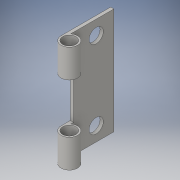
# Autodesk Inventor part: Hinge Wall 1
Saved by Autodesk Inventor 2016 (Build 200138000, 138)
## iProperties
Created: 2016-04-01
Part Number: Hinge Wall 1
Material: Generic
Document SubType Name: Modeling
Designer: amycroft3
Density: 1 g/cm^3
Appearance: Default
Author: amycroft3
Autodesk Inventor part; units mm, degrees
ref_plane "YZ Plane" through (0, 0, 0) normal (1, 0, 0) x (0, 1, 0)
ref_plane "XY Plane" through (0, 0, 0) normal (0, 0, 1) x (1, 0, 0)
sketch "Sketch1" plane through (0, 0, 0) normal (0, 1, 0) x (-1, 0, 0)
  circle A0 centre (0, 0) radius 2.3876
  arc A1 (2.9591, 0) -> (1.8161, -2.3362) centre (0, 0) ccw
  line L0 (2.9591, 0) -> (2.3876, 0)
  line L1 (1.8161, -2.3362) -> (1.8161, -17.78)
  line L2 (1.8161, -17.78) -> (2.9591, -17.78)
  line L3 (2.9591, -17.78) -> (2.9591, 0)
  dimension "d0" = 4.7752
  dimension "d1" = 5.9182
  dimension "d2" = 17.78
  dimension "d3" = 1.143
  constraints: 8 end point, 2 coincident, 2 parallel, 2 point on circle, 1 centre point, 1 horizontal, 1 horizontal alignment, 1 perpendicular, 1 tangent, 2 other
  measures "d1" diameter of A1
  measures "d2" distance of L2.end L0.start
  measures "d3" distance of L1.end L2.end
extrude "Extrusion1" add sketch "Sketch1" along normal blind 38.1
ref_plane "Work Plane1" through (0, 10.16, 0) normal (0, 1, 0) x (-1, 0, 0)
sketch "Sketch2" plane through (0, 10.16, 0) normal (0, 1, 0) x (-1, 0, 0)
  circle A0 centre (0, 0) radius 2.3876 projected
  arc A1 (2.9591, 0) -> (1.8161, -2.3362) centre (0, 0) ccw projected
  line L0 (1.8161, -2.3362) -> (1.8161, -17.78) projected
  line L1 (1.8161, -17.78) -> (2.9591, -17.78) projected
  line L2 (2.9591, -17.78) -> (2.9591, 0) projected
  line L3 (2.9591, 3.4646) -> (-3.1409, 3.4646)
  line L4 (-3.1409, 3.4646) -> (-3.1409, -3.337)
  line L5 (-3.1409, -3.337) -> (2.9591, -3.337)
  line L6 (2.9591, -3.337) -> (2.9591, 3.4646)
  dimension "d7" = 0
  dimension "d8" = 6.1
  dimension "d9" = 21.2446
  dimension "d10" = 14.443
  constraints: 8 end point, 2 parallel, 1 horizontal, 1 perpendicular
  measures "d7" distance between parallel lines of L2 L6
  measures "d8" distance between parallel lines of L2 L4
  measures "d9" distance between parallel lines of L1 L3
  measures "d10" distance between parallel lines of L1 L5
extrude "Extrusion2" cut sketch "Sketch2" along normal blind 17.78 contours L2 L5 L0 A1 | A1 L0 L5 L4 L3 L6
sketch "Sketch3" plane through (-1.8161, 0, -2.3362) normal (1, 0, 0) x (0, 0, -1)
  circle A0 centre (9.0938, 5.08) radius 2.54
  circle A1 centre (9.0938, 33.02) radius 2.54
  line L0 (15.4438, 0) -> (15.4438, 38.1) projected
  line L1 (0, 0) -> (15.4438, 0) projected
  line L2 (0, 38.1) -> (15.4438, 38.1) projected
  point P0 (-2.3362, 0)
  dimension "d13" = 6.35
  dimension "d14" = 5.08
  dimension "d15" = 5.08
  dimension "d17" = 5.08
  constraints: 2 centre point, 1 equal radius, 1 vertical alignment
  measures "d13" distance from line of A0.centre L0
  measures "d14" distance from line of A0.centre L1
  measures "d15" diameter of A0
  measures "d17" distance from line of A1.centre L2
extrude "Extrusion3" cut sketch "Sketch3" against normal up to next
equation "\"d17\" = d14"
body "Solid1"
